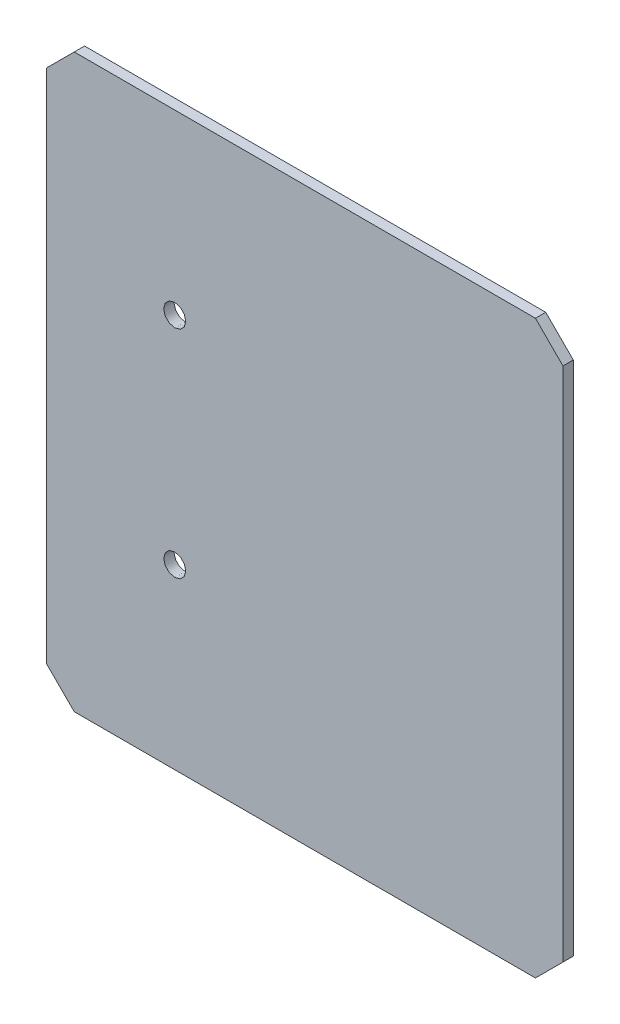
# Autodesk Inventor part: power_board
Saved by Autodesk Inventor 2025 (Build 290162000, 162)
## iProperties
Created: 2026-08-11
Part Number: power_board
Material: Типовые
Document SubType Name: Modeling
Designer: garin
Density: 1 g/cm^3
Appearance: По умолчанию
Author: garin
Autodesk Inventor part; units mm, degrees
ref_plane "YZ Plane" through (0, 0, 0) normal (1, 0, 0) x (0, 1, 0)
ref_plane "XZ Plane" through (0, 0, 0) normal (0, 1, 0) x (-1, 0, 0)
ref_plane "XY Plane" through (0, 0, 0) normal (0, 0, 1) x (1, 0, 0)
sketch "Эскиз1" plane through (0, 0, 0) normal (0, 0, 1) x (1, 0, 0)
  line L0 (-30, 41.5) -> (26, 41.5)
  line L1 (30, 37.5) -> (30, -37.5)
  line L2 (26, -41.5) -> (-30, -41.5)
  line L3 (-30, -41.5) -> (-30, 41.5)
  line L4 (-30, 41.5) -> (30, -41.5) construction
  line L5 (30, 41.5) -> (-30, -41.5) construction
  line L6 (-30, -41.5) -> (-41, -41.5)
  line L7 (-45, -37.5) -> (-45, 37.5)
  line L8 (-41, 41.5) -> (-30, 41.5)
  line L9 (-30, 41.5) -> (-30, -41.5)
  line L10 (-41, -41.5) -> (-45, -37.5)
  line L11 (-45, 37.5) -> (-41, 41.5)
  line L12 (26, 41.5) -> (30, 37.5)
  line L13 (26, -41.5) -> (30, -37.5)
  line L14 (0, 0) -> (-26.4, 0) construction
  line L15 (-26.4, 0) -> (-26.4, 15.7) construction
  line L16 (-26.4, 15.7) -> (0, 15.7) construction
  line L17 (0, 15.7) -> (0, 0) construction
  circle A0 centre (-26.4, 15.7) radius 1.6
  circle A1 centre (-26.4, -15.7) radius 1.6
  circle A2 centre (26.4, 15.7) radius 1.6
  circle A3 centre (26.4, -15.7) radius 1.6
  point P0 (-45, 41.5)
  point P1 (-45, -41.5)
  dimension "d0" = 60
  dimension "d1" = 83
  dimension "d2" = 15
  dimension "d3" = 83
  dimension "d6" = 4
  dimension "d7" = 4
  dimension "d8" = 4
  dimension "d9" = 4
  dimension "d10" = 4
  dimension "d11" = 4
  dimension "d12" = 4
  dimension "d13" = 4
  dimension "d14" = 26.4
  dimension "d15" = 15.7
  dimension "d16" = 3.2
  constraints: 36 end point, 8 point on line, 6 parallel, 4 centre point, 3 horizontal, 3 perpendicular, 3 symmetric about line, 2 midpoint, 1 coincident, 3 other
  measures "d0" distance of L4.end L2.end
  measures "d1" distance of L5.start L4.end
  measures "d2" distance of point (-45, 41.5) L8.end
  measures "d3" distance of point (-45, -41.5) point (-45, 41.5)
  measures "d6" distance of L6.end point (-45, -41.5)
  measures "d7" distance of L7.start point (-45, -41.5)
  measures "d8" distance of L7.end point (-45, 41.5)
  measures "d9" distance of L8.start point (-45, 41.5)
  measures "d10" distance of L0.end L5.start
  measures "d11" distance of L1.start L5.start
  measures "d12" distance of L2.start L4.end
  measures "d13" distance of L1.end L4.end
  measures "d14" distance of L15.end L16.end
  measures "d15" distance of L14.end L15.end
  measures "d16" diameter of A0
extrude "Выдавливание1" add sketch "Эскиз1" along normal blind 1.5 contours L0 L12 L1 L13 L2 L3 | L3 L6 L10 L7 L11 L8 | A2 | A3
equation "\"d7\" = d6"
equation "\"d9\" = d8"
equation "\"d10\" = d6"
equation "\"d11\" = d10"
